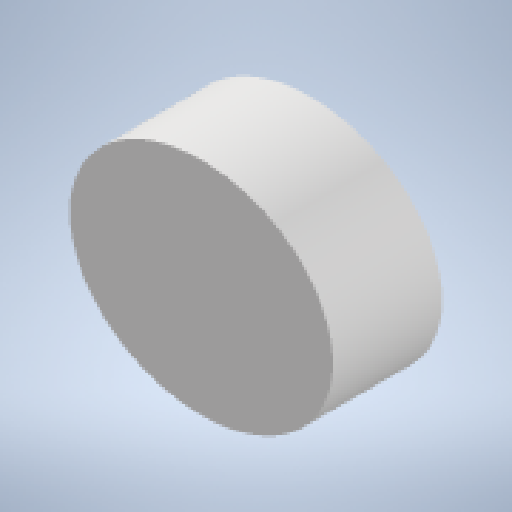
# Autodesk Inventor part: LeftCheekPeach
Saved by Autodesk Inventor 2023 (Build 270158000, 158)
## iProperties
Created: 2022-11-09
Part Number: LeftCheekPeach
Material: Generic
Document SubType Name: Modeling
Designer: reide
Density: 1 g/cm^3
Appearance: Default
Author: reide
Autodesk Inventor part; units mm, degrees
ref_plane "YZ Plane" through (0, 0, 0) normal (1, 0, 0) x (0, 1, 0)
ref_plane "XZ Plane" through (0, 0, 0) normal (0, 1, 0) x (-1, 0, 0)
ref_plane "XY Plane" through (0, 0, 0) normal (0, 0, 1) x (1, 0, 0)
sketch "Sketch1" plane through (0, 0, 0) normal (0, 0, 1) x (1, 0, 0)
  arc A0 (-9.1161, 25.7586) -> (-13.313, 21.8774) centre (-8.2115, 20.5707) ccw projected
  ellipse E0 centre (-18.0763, 22.3083) end of major axis (-22.8397, 22.7393) minor radius 4.1297 (-13.4391, 21.2064) -> (-13.313, 21.8774) ccw projected
  arc A1 (-13.313, 21.8774) -> (-13.4391, 21.2064) centre (-8.2115, 20.5707) ccw projected
  ellipse E1 centre (-18.0763, 22.3083) end of major axis (-13.313, 21.8774) minor radius 4.1297 (-13.313, 21.8774) -> (-15.5486, 25.7586) ccw projected
  line L0 (-9.1161, 25.7586) -> (-15.5486, 25.7586) projected
  arc A2 (-67.787, 25.7586) -> (-69.1237, 23.7196) centre (-50.5026, 12.9698) ccw projected
  spline S0 degree 3 poles (-65.1091, 22.0003) (-65.1168, 21.9714) (-65.1247, 21.9426) (-65.2552, 21.496) (-65.4592, 21.1022) (-65.9414, 20.4921) (-66.1949, 20.2555) (-66.7389, 19.9003) (-67.0236, 19.7722) (-67.5793, 19.6428) (-67.8465, 19.6266) (-68.2695, 19.6888) (-68.4292, 19.734) (-68.5796, 19.8005) (-68.8638, 19.9261) (-69.1122, 20.1291) (-69.4038, 20.5184) (-69.4901, 20.673) (-69.7149, 21.2159) (-69.768, 21.6358) (-69.6981, 22.5727) (-69.5232, 23.0866) (-69.2071, 23.5982) (-69.1664, 23.6596) (-69.1237, 23.7196) knots -2.04297 -2.04297 -2.04297 -2.04297 -2.033998 -2.033998 -1.903383 -1.903383 -1.8007 -1.8007 -1.70847 -1.70847 -1.629539 -1.629539 -1.580207 -1.580207 -1.580207 -1.486994 -1.486994 -1.434286 -1.434286 -1.31073 -1.31073 -1.152429 -1.152429 -1.130329 -1.130329 -1.130329 -1.130329 projected
  arc A3 (-62.2466, 25.7586) -> (-65.1091, 22.0003) centre (-57.3704, 19.0752) ccw projected
  line L1 (-57.002, 25.7586) -> (-62.2466, 25.7586) projected
  arc A4 (-57.002, 25.7586) -> (-52.5716, 21.9614) centre (-43.5692, 36.9484) ccw projected
  arc A5 (-52.5716, 21.9614) -> (-61.5285, 13.9346) centre (-49.152, 9.1347) ccw projected
  arc A6 (-61.5285, 13.9346) -> (-63.3685, -3.1136) centre (-33.7061, 2.3083) ccw projected
  arc A7 (-63.3685, -3.1136) -> (-70.3816, -14.3561) centre (-52.3561, -17.7917) ccw projected
  arc A8 (-70.3816, -14.3561) -> (-57.0518, -18.6263) centre (-59.4561, -3.1917) ccw projected
  arc A9 (-57.0518, -18.6263) -> (-11.4801, -27.2893) centre (-28.9353, 5.0839) ccw projected
  arc A10 (-11.4801, -27.2893) -> (1.6202, -27.979) centre (-4.1305, -12.4483) ccw projected
  arc A11 (1.6202, -27.979) -> (-1.176, -17.8593) centre (-12.997, -26.5718) ccw projected
  arc A12 (-1.176, -17.8593) -> (1.4991, -4.3136) centre (-20.384, -7.0289) ccw projected
  arc A13 (1.4991, -4.3136) -> (-5.025, 17.7342) centre (-8.2115, 4.8022) ccw projected
  arc A14 (-5.025, 17.7342) -> (-7.398, 24.7586) centre (-8.2115, 20.5707) ccw projected
  line L2 (-7.398, 24.7586) -> (-6.0187, 24.7586) projected
  arc A15 (-5.0187, 25.7586) -> (-6.0187, 24.7586) centre (-5.0187, 24.7586) ccw projected
  line L3 (62.1444, 25.7586) -> (-5.0187, 25.7586) projected
  line L4 (62.1444, 33.7601) -> (62.1444, 25.7586) projected
  line L5 (-69.6317, 33.7601) -> (62.1444, 33.7601) projected
  arc A16 (-71.6317, 35.7601) -> (-69.6317, 33.7601) centre (-69.6317, 35.7601) ccw projected
  line L6 (-71.6317, 128.7586) -> (-71.6317, 35.7601) projected
  arc A17 (-69.6317, 130.7586) -> (-71.6317, 128.7586) centre (-69.6317, 128.7586) ccw projected
  line L7 (62.1444, 130.7586) -> (-69.6317, 130.7586) projected
  line L8 (62.1444, 138.7586) -> (62.1444, 130.7586) projected
  line L9 (-75.0567, 138.7586) -> (62.1444, 138.7586) projected
  arc A18 (-75.0567, 138.7586) -> (-79.0567, 134.7586) centre (-75.0567, 134.7586) ccw projected
  line L10 (-79.0567, 29.7586) -> (-79.0567, 134.7586) projected
  arc A19 (-79.0567, 29.7586) -> (-75.0567, 25.7586) centre (-75.0567, 29.7586) ccw projected
  line L11 (-67.787, 25.7586) -> (-75.0567, 25.7586) projected
  ellipse E2 centre (-18.8703, 22.3083) end of major axis (-23.3081, 22.3083) minor radius 3.9921 projected
  ellipse E3 centre (-35.4561, 3.2586) end of major axis (-38.4561, 3.2586) minor radius 2.4928 projected
  arc A20 (-62.6379, -4.8899) -> (-58.0267, -16.7499) centre (77.4596, 42.753) ccw projected
  arc A21 (-68.1575, -13.5015) -> (-58.0267, -16.7499) centre (-57.4866, 2.3559) ccw projected
  arc A22 (-62.6379, -4.8899) -> (-68.1575, -13.5015) centre (-49.6205, -19.308) ccw projected
  arc A23 (-13.852, 0.2906) -> (-15.4561, -0.7414) centre (-14.0803, -1.1173) ccw projected
  arc A24 (-15.4561, -0.7414) -> (-17.3822, 1.2329) centre (-18.4561, -1.7414) ccw projected
  ellipse E4 centre (-15.612, 1.2586) end of major axis (-15.612, 10.2586) minor radius 1.7702 (-13.852, 0.2906) -> (-17.3822, 1.2329) ccw projected
  circle A25 centre (-6.4561, -3.1917) radius 2.7388 projected
  circle A26 centre (-28.4561, -1.7414) radius 2.8284 projected
  arc A27 (-7.2787, -26.7401) -> (-0.9865, -20.9367) centre (-21.6094, -4.8899) ccw projected
  arc A28 (-0.5284, -26.6587) -> (-0.9865, -20.9367) centre (-18.722, -25.2361) ccw projected
  arc A29 (-7.2787, -26.7401) -> (-0.5284, -26.6587) centre (-4.0898, -11.2585) ccw projected
  ellipse E5 centre (-8.2115, 20.8216) end of major axis (-4.1929, 20.5457) minor radius 3.5714 projected
  ellipse E6 centre (0, 0) end of major axis (-2.5315, 0) minor radius 2.1289 projected
  ellipse E7 centre (0, 0) end of major axis (2.4049, 0) minor radius 2.0224
  constraints: 1 centre point, 1 coincident, 7 other
extrude "Extrusion1" add sketch "Sketch1" along normal blind 2 contours E7
body "Solid1"
